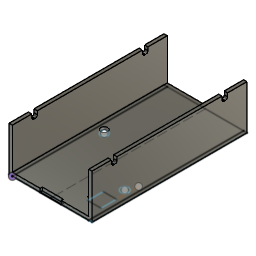
Cover_V2 (Autodesk Fusion 360 design; units mm, degrees)
part number: 2025-10-18-14-32-01-691
Autodesk Fusion 360 part; units mm, degrees
sketch "Sketch1" plane through (0, 0, 0) normal (0, 0, 1) x (1, 0, 0)
  line L0 (0, 0) -> (69, 0)
  line L1 (69, 0) -> (69, 140)
  line L2 (69, 140) -> (0, 140)
  line L3 (0, 140) -> (0, 0)
  line L4 (0, 140) -> (-3, 140)
  line L5 (-3, 140) -> (-3, 0)
  line L6 (-3, 0) -> (0, 0)
  line L7 (0, 0) -> (0, 140)
  line L8 (69, 140) -> (72, 140)
  line L9 (72, 140) -> (72, 0)
  line L10 (72, 0) -> (69, 0)
  line L11 (69, 0) -> (69, 140)
  line L12 (34.5, 140) -> (34.5, 0) construction
  line L13 (25, 0) -> (44, 0)
  line L14 (44, 0) -> (44, 2)
  line L15 (44, 2) -> (25, 2)
  line L16 (25, 2) -> (25, 0)
  line L17 (34.5, 2) -> (34.5, 0) construction
  line L18 (53.1198, 29) -> (65.1198, 29)
  line L19 (65.1198, 29) -> (65.1198, 15)
  line L20 (65.1198, 15) -> (53.1198, 15)
  line L21 (53.1198, 15) -> (53.1198, 29)
  circle A0 centre (8, 75) radius 3.175
  circle A1 centre (61.6198, 40) radius 3.5
  line L22 (65.1198, 29) -> (65.1198, 49) construction
  dimension "d1" = 140
  dimension "d3" = 3
  dimension "d4" = 3
  dimension "d30" = 75
  dimension "d31" = 2
  dimension "d32" = 19
  dimension "d33" = 14
  dimension "d34" = 12
  dimension "d35" = 6.35
  dimension "d36" = 65
  dimension "d37" = 7
  dimension "d38" = 40
  dimension "d39" = 15
  constraint horizontal L0
  constraint vertical L1
  constraint horizontal L2
  constraint vertical L3
  constraint coincident L0.start L3.end
  constraint horizontal L4
  constraint vertical L5
  constraint horizontal L6
  constraint vertical L7
  constraint horizontal L8
  constraint vertical L9
  constraint horizontal L10
  constraint vertical L11
  constraint midpoint L2 L12.start
  constraint midpoint L0 L12.end
  constraint horizontal L13
  constraint vertical L14
  constraint horizontal L15
  constraint vertical L16
  constraint coincident L0 L13.start
  constraint midpoint L15 L17.start
  constraint midpoint L13 L12.end
  constraint coincident L12 L17.start
  constraint horizontal L18
  constraint vertical L19
  constraint horizontal L20
  constraint vertical L21
  constraint perpendicular L18 L22
  constraint tangent A1 L22
  measures "d1" distance of L0.start L2.end
  measures "d3" distance of L5 L7
  measures "d4" distance of L9 L11
  measures "d30" distance of L5 L9
  measures "d31" distance of L13.start L15.end
  measures "d32" distance of L14 L16
  measures "d33" distance of L18.start L20.end
  measures "d34" distance of L19 L21
  measures "d35" diameter of A0
  measures "d36" distance of L2 A0.centre
  measures "d37" diameter of A1
  measures "d38" distance of L0 A1.centre
  measures "d39" distance of L0 L20
extrude "Extrude1" add sketch "Sketch1" along normal blind 3 contours L0 L1 L2 L3 L7 L11 L14 L15 L16
extrude "Extrude2" add sketch "Sketch1" along normal blind 40 contours L3 L4 L5 L6 L7 | L1 L8 L9 L10 L11
sketch "Sketch3" plane through (72, 0, 0) normal (1, 0, 0) x (0, 1, 0)
  line L0 (0, 0) -> (140, 0)
  line L1 (140, 0) -> (140, 40)
  line L2 (140, 40) -> (0, 40)
  line L3 (0, 40) -> (0, 0)
  line L4 (140, 0) -> (0, 0)
  line L5 (70, 40) -> (70, 0) construction
  line L6 (17.5, 40) -> (22.5, 40)
  line L7 (22.5, 40) -> (22.5, 37)
  line L8 (20.5, 35) -> (19.5, 35)
  line L9 (17.5, 37) -> (17.5, 40)
  arc A0 (17.5, 37) -> (19.5, 35) centre (19.5, 37) ccw
  arc A1 (20.5, 35) -> (22.5, 37) centre (20.5, 37) ccw
  line L10 (20, 40) -> (20, 35) construction
  line L11 (117.5, 40) -> (122.5, 40)
  line L12 (122.5, 40) -> (122.5, 37)
  line L13 (120.5, 35) -> (119.5, 35)
  line L14 (117.5, 37) -> (117.5, 40)
  arc A2 (117.5, 37) -> (119.5, 35) centre (119.5, 37) ccw
  arc A3 (120.5, 35) -> (122.5, 37) centre (120.5, 37) ccw
  line L15 (120, 35) -> (120, 40) construction
  point P0 (17.5, 35)
  point P1 (117.5, 35)
  dimension "d18" = 5
  dimension "d19" = 5
  dimension "d20" = 2
  dimension "d21" = 2
  dimension "d23" = 5
  dimension "d24" = 2
  dimension "d25" = 2
  dimension "d26" = 5
  dimension "d27" = 100
  constraint midpoint L2 L5.start
  constraint midpoint L4 L5.end
  constraint horizontal L6
  constraint vertical L7
  constraint horizontal L8
  constraint vertical L9
  constraint coincident L2 L6.start
  constraint coincident P0 L8
  constraint coincident P0 L9
  constraint tangent L8 A0
  constraint tangent L9 A0
  constraint tangent L7 A1
  constraint tangent L8 A1
  constraint midpoint L6 L10.start
  constraint midpoint L8 L10.end
  constraint horizontal L11
  constraint vertical L12
  constraint horizontal L13
  constraint vertical L14
  constraint coincident L2 L11.start
  constraint coincident P1 L13
  constraint coincident P1 L14
  constraint tangent L13 A2
  constraint tangent L14 A2
  constraint tangent L12 A3
  constraint tangent L13 A3
  constraint midpoint L13 L15.start
  constraint midpoint L11 L15.end
  constraint symmetric L5 L10 L15
  measures "d18" distance of L6.start P0
  measures "d19" distance of L7 L9
  measures "d20" radius of A0
  measures "d21" radius of A1
  measures "d23" distance of L12 L14
  measures "d24" radius of A2
  measures "d25" radius of A3
  measures "d26" distance of L11 L13
  measures "d27" distance of L10 L15
extrude "Extrude3" cut sketch "Sketch3" along normal mid plane 200 contours L2 L6 L7 L8 L9 A0 A1 | L2 L11 L12 L13 L14 A2 A3
